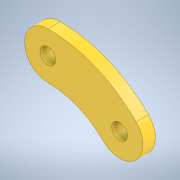
# Autodesk Inventor part: Support
Saved by Autodesk Inventor 2020.3 (Build 243373000, 373)
## iProperties
Created: 2021-06-11
Part Number: Support
Material: Steel, Mild
Document SubType Name: Modeling
Designer: User
Density: 7.85 g/cm^3
Appearance: Glossy - Gold
Mass: 129.685 g
Surface Area: 62.1986 cm^2
Volume: 16.5204 cm^3
Author: User
Autodesk Inventor part; units mm, degrees
ref_plane "YZ Plane" through (0, 0, 0) normal (1, 0, 0) x (0, 1, 0)
ref_plane "XZ Plane" through (0, 0, 0) normal (0, 1, 0) x (-1, 0, 0)
ref_plane "XY Plane" through (0, 0, 0) normal (0, 0, 1) x (1, 0, 0)
sketch "Sketch1" plane through (0, 0, 0) normal (0, 0, 1) x (1, 0, 0)
  arc A0 (45.9619, 45.9619) -> (0, 65) centre (0, 0) ccw construction
  arc A1 (56.5685, 56.5685) -> (0, 80) centre (0, 0) ccw
  arc A2 (35.3553, 35.3553) -> (0, 50) centre (0, 0) ccw
  arc A3 (35.3553, 35.3553) -> (56.5685, 56.5685) centre (45.9619, 45.9619) ccw
  arc A4 (0, 80) -> (0, 50) centre (0, 65) ccw
  line L0 (0, 65) -> (0, 0)
  line L1 (0, 0) -> (45.9619, 45.9619)
  circle A5 centre (0, 65) radius 5
  circle A6 centre (45.9619, 45.9619) radius 5
  dimension "d0" = 45
  dimension "d1" = 50
  dimension "d2" = 80
  dimension "d3" = 10
  dimension "d4" = 10
  constraints: 10 point on circle, 7 centre point, 4 end point, 4 tangent, 3 coincident, 1 vertical
  measures "d0" angle of L0 L1
  measures "d1" radius of A2
  measures "d2" radius of A1
  measures "d3" diameter of A5
  measures "d4" diameter of A6
extrude "Extrusion1" add sketch "Sketch1" along normal blind 7.9375 contours A3 A2 A4 A1
body "Solid1"
